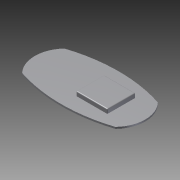
# Autodesk Inventor part: Bluetooth
Saved by Autodesk Inventor 2012 (Build 160160000, 160)
## iProperties
Created: 2016-11-08
Part Number: Bluetooth
Material: Default
Document SubType Name: Modeling
Designer: EGarcia
Density: 1 g/cm^3
Author: EGarcia
Autodesk Inventor part; units mm, degrees
ref_plane "YZ Plane" through (0, 0, 0) normal (1, 0, 0) x (0, 1, 0)
ref_plane "XZ Plane" through (0, 0, 0) normal (0, 1, 0) x (-1, 0, 0)
ref_plane "XY Plane" through (0, 0, 0) normal (0, 0, 1) x (1, 0, 0)
sketch "Boceto1" plane through (0, 0, 0) normal (0, 0, 1) x (1, 0, 0)
  arc A0 (60, 29.35) -> (32.5, 33.7) centre (32.5, -55.4003) ccw
  arc A1 (32.5, 33.7) -> (5, 29.35) centre (32.5, -55.4003) ccw
  arc A2 (32.5, 0) -> (60, 4.35) centre (32.5, 89.1003) ccw
  arc A3 (60, 4.35) -> (60, 29.35) centre (46.875, 16.85) ccw
  arc A4 (5, 4.35) -> (32.5, 0) centre (32.5, 89.1003) ccw
  arc A5 (5, 29.35) -> (5, 4.35) centre (18.125, 16.85) ccw
  line L0 (32.5, 16.85) -> (32.5, 8.6)
  line L1 (32.5, 8.6) -> (32.5, 25.1)
  line L2 (32.5, 25.1) -> (51, 25.1)
  line L3 (51, 25.1) -> (51, 8.6)
  line L4 (51, 8.6) -> (32.5, 8.6)
  line L5 (32.5, 8.6) -> (32.5, 25.1)
  point P0 (0, 0)
  dimension "d6" = 8.25
  dimension "d7" = 16.5
  constraints: 12 end point, 12 point on circle, 6 centre point, 2 parallel, 1 horizontal, 1 midpoint, 1 perpendicular
  measures "d6" distance of L0.start L0.end
  measures "d7" distance of L0.end L1.end
extrude "Extrusión1" add sketch "Boceto1" along normal blind 2.5 and the other way blind 1 contours L1 L2 L3 L4 L0
extrude "Extrusión2" add sketch "Boceto1" against normal blind 1
sketch "Boceto2" plane through (0, 0, -1) normal (0, 0, -1) x (-1, 0, 0)
  arc A0 (-5, 4.35) -> (-5, 29.35) centre (-18.125, 16.85) ccw projected
  line L0 (0, 16.85) -> (-5, 16.85)
  line L1 (-5, 16.85) -> (-5, 13.85)
  line L2 (-5, 13.85) -> (-14.5, 13.85)
  line L3 (-14.5, 13.85) -> (-14.5, 7.85)
  line L4 (-14.5, 7.85) -> (-5, 7.85)
  line L5 (-5, 7.85) -> (-5, 13.85)
  line L6 (-5, 13.85) -> (-14.5, 13.85)
  line L7 (-14.5, 13.85) -> (-14.5, 7.85)
  point P0 (0, 0)
  dimension "d14" = 5
  dimension "d15" = 3
  dimension "d16" = 9.5
  dimension "d18" = 6
  constraints: 16 end point, 3 parallel, 3 perpendicular, 2 horizontal, 1 point on circle
  measures "d14" distance of L0.start L0.end
  measures "d15" distance of L0.end L1.end
  measures "d16" distance of L1.end L2.end
  measures "d18" distance of L2.end L3.end
extrude "Extrusión3" add sketch "Boceto2" along normal blind 3.8
fillet "Empalme1" radius 0.5 16 edges at (5, 13.85, -2.9) (14.5, 13.85, -2.9) (9.75, 13.85, -4.8) (9.75, 7.85, -4.8) (14.5, 10.85, -4.8) (5, 10.85, -4.8) (41.75, 25.1, 2.5) (51, 16.85, 2.5) (41.75, 8.6, 2.5) (32.5, 16.85, 2.5) (32.5, 25.1, 1.25) (51, 25.1, 1.25) (32.5, 8.6, 1.25) (51, 8.6, 1.25) (5, 7.85, -2.9) (14.5, 7.85, -2.9)
